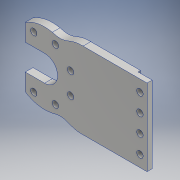
# Autodesk Inventor part: test_side_u64
Saved by Autodesk Inventor 2018 (Build 220112000, 112)
## iProperties
Created: 2016-12-19
Part Number: test_side_u64
Material: Aluminum 6061
Document SubType Name: Modeling
Designer: steve
Density: 2.7 g/cm^3
Appearance: Aluminum - Flat
Mass: 8.1898 g
Surface Area: 28.0523 cm^2
Volume: 3.03326 cm^3
Vendor: Rhoban
d13: 3,000 mm
d14: 6,000 mm
d0: 30,000 mm
d1: 22,000 mm
d2: 40,000 mm
d3: 10,100 mm
d4: 30,000 mm
d5: 28,000 mm
d6: 15,000 mm
d7: 12,000 mm
d8: 2,500 mm
d15: 3,000 mm
d16: 0,00 deg
d18: 6,000 ul
d19: 22,000 mm
d20: 225,00 deg
d22: 2,500 mm
d29: 3,000 mm
d30: 4,500 mm
d31: 4,000 ul
d33: 7,000 mm
d38: 2,500 mm
d47: 5,500 mm
d48: 1,000 mm
d49: 0,00 deg
d50: 3,100 mm
d51: 2,500 mm
d52: 1,000 mm
d53: 0,00 deg
d54: 1,500 mm
d55: 30,000 mm
d56: 7,000 mm
d57: 7,000 mm
d58: 7,000 mm
d59: 4,500 mm
d61: 2,500 mm
d68: 22,50 deg
d9: 30,000 mm
d10: 22,000 mm
d11: 21,000 mm
horn_radius_clearance: 10,100 mm
d21: 22,000 mm
d60: 4,500 mm
Author: steve
Autodesk Inventor part; units mm, degrees
ref_plane "YZ Plane" through (0, 0, 0) normal (1, 0, 0) x (0, 1, 0)
ref_plane "XZ Plane" through (0, 0, 0) normal (0, 1, 0) x (-1, 0, 0)
sketch "Sketch1" plane through (0, 0, 0) normal (0, 1, 0) x (-1, 0, 0)
  line L0 (-40, 15) -> (0, 15) construction
  line L1 (15, 15) -> (15, -15) construction
  line L2 (15, -15) -> (0, -15) construction
  line L3 (-40, -15) -> (-40, 15)
  line L4 (15, 0) -> (-40, 0) construction
  line L5 (-28.4, 0) -> (23.4, 0) construction
  circle A0 centre (0, 0) radius 11 construction
  line L6 (11, 15) -> (11, -15) construction
  circle A1 centre (0, 0) radius 5.05 construction
  line L7 (0, 5.05) -> (7.55, 5.05) construction
  line L8 (0, -5.05) -> (7.55, -5.05) construction
  line L9 (15, 15) -> (15, 5) construction
  line L10 (15, -5) -> (15, -15) construction
  arc A2 (0, 5.05) -> (0, -5.05) centre (0, 0) ccw
  circle A3 centre (0, 0) radius 15 construction
  arc A4 (0, -15) -> (14.1421, -5) centre (0, 0) ccw construction
  arc A5 (14.1421, 5) -> (0, 15) centre (0, 0) ccw construction
  line L11 (0, -15) -> (-40, -15) construction
  line L12 (0, 15) -> (15, 15) construction
  arc A6 (11, -8.6603) -> (11, 8.6603) centre (0, 0) ccw construction
  line L13 (-3, -15) -> (-3, 15) construction
  arc A7 (-3, -13.6748) -> (7.55, -11.7897) centre (0, 0) ccw
  line L14 (7.55, 5.05) -> (0, 5.05)
  line L15 (-15, -18.6523) -> (-15, 18.2394) construction
  line L16 (-40, -15) -> (-15, -15)
  line L17 (-40, 15) -> (-15, 15)
  spline S0 degree 4 poles (-3, -13.6748) (-4.5129, -13.3429) (-7.4407, -12.2328) (-10.459, -15) (-13.4863, -15) (-15, -15) knots 0 0 0 0 0 0.5 1 1 1 1 1
  spline S1 degree 4 poles (-3, 13.6748) (-4.5129, 13.3429) (-7.4407, 12.2328) (-10.459, 15) (-13.4863, 15) (-15, 15) knots 0 0 0 0 0 0.5 1 1 1 1 1
  line L18 (5.05, -15) -> (5.05, 15) construction
  line L19 (7.55, -11.7897) -> (7.55, -5.05)
  line L20 (7.55, 5.05) -> (7.55, 11.7897)
  line L21 (7.55, -5.05) -> (11, -5.05) construction
  line L22 (7.55, 5.05) -> (9.7723, 5.05) construction
  arc A8 (7.55, 11.7897) -> (7.55, -11.7897) centre (0, 0) ccw construction
  arc A9 (7.55, 11.7897) -> (-3, 13.6748) centre (0, 0) ccw
  line L23 (0, -5.05) -> (7.55, -5.05)
  line L24 (0, -26.0306) -> (0, 25.6178) construction
  line L25 (35.28, 0) -> (-47.88, 0) construction
  point P0 (13.0767, -5)
  dimension "d1" = 22
  dimension "d0" = 30
  dimension "d2" = 40
  dimension "d3" = 10.1
  dimension "d4" = 30
  dimension "d5" = 28
  dimension "d6" = 15
  dimension "d7" = 12
  dimension "d8" = 2.5
  constraints: 48 end point, 20 point on circle, 20 point on line, 9 centre point, 8 coincident, 6 collinear, 6 horizontal, 6 perpendicular, 5 parallel, 5 tangent, 5 vertical, 2 midpoint, 8 other
  measures "d0" distance of L9.start L2.start
  measures "d2" distance from line of point (0, 0) L3
  measures "d3" diameter of A1
  measures "d4" diameter of A3
  measures "d5" diameter of A6
  measures "d6" distance from line of L15 point (0, 0)
  measures "d7" distance between parallel lines of L13 L15
  measures "d8" distance between parallel lines of L19 L18
extrude "Extrusion1" add sketch "Sketch1" along normal blind 3
sketch "Sketch2" plane through (0, 3, 0) normal (0, 1, 0) x (1, 0, 0)
  circle A0 centre (0, 0) radius 11 construction
  line L0 (-21.2, 0) -> (50.2, 0) construction
  line L1 (0, 21) -> (0, -21) construction
  line L2 (0, 0) -> (-4.2095, -10.1627) construction
  point P0 (-4.2095, -10.1627)
  point P1 (4.2095, -10.1627)
  point P2 (10.1627, -4.2095)
  point P3 (10.1627, 4.2095)
  point P4 (4.2095, 10.1627)
  point P5 (-4.2095, 10.1627)
  dimension "d19" = 22
  dimension "d20" = 225
  dimension "d68" = 22.5
  constraints: 3 coincident, 2 end point, 2 point on circle, 1 centre point, 6 other
  measures "d19" diameter of A0
  measures "d68" angle of L1 L2
hole "Hole1" at (-4.2095, 3, 10.1627) at (-4.2095, 3, -10.1627) at (4.2095, 3, -10.1627) at (10.1627, 3, -4.2095) at (10.1627, 3, 4.2095) at (4.2095, 3, 10.1627) direction (0, -1, 0) diameter 2.5 end through all
sketch "Sketch3" plane through (0, 3, 0) normal (0, 1, 0) x (1, 0, 0)
  circle A0 centre (-4.2095, -10.1627) radius 1.25 construction
  circle A1 centre (4.2095, -10.1627) radius 1.25 construction
  circle A2 centre (10.1627, -4.2095) radius 1.25 construction
  circle A3 centre (10.1627, 4.2095) radius 1.25 construction
  circle A4 centre (4.2095, 10.1627) radius 1.25 construction
  circle A5 centre (-4.2095, 10.1627) radius 1.25 construction
  point P0 (0, 0)
sketch "Sketch4" plane through (0, 3, 0) normal (0, 1, 0) x (1, 0, 0)
  line L0 (37, -21.9283) -> (37, 20.7608) construction
  line L1 (40, -15) -> (40, 15) construction
  line L2 (15, -15) -> (40, -15) construction
  point P0 (0, 0)
  point P1 (37, -10.5)
  point P2 (37, -3.5)
  point P3 (37, 3.5)
  point P4 (37, 10.5)
  dimension "d29" = 3
  dimension "d30" = 4.5
  dimension "d33" = 7
  constraints: 2 end point, 2 vertical, 1 point on line, 3 other
  measures "d29" distance between parallel lines of L1 L0
  measures "d30" distance from line of L2 point (37, -10.5)
  measures "d33" distance of point (37, -10.5) point (37, -3.5)
hole "Hole2" [suppressed]
sketch "Sketch6" plane through (0, 3, 0) normal (0, 1, 0) x (1, 0, 0)
  line L0 (15, -15) -> (40, -15) projected
  line L1 (40, -15) -> (34.5, -15)
  line L2 (34.5, -15) -> (34.5, 15)
  line L3 (34.5, 15) -> (40, 15)
  line L4 (40, 15) -> (40, -15)
  line L5 (37.25, 15) -> (37.25, -15) construction
  point P0 (0, 0)
  point P1 (37.25, -10.5)
  point P2 (37.25, -3.5)
  point P3 (37.25, 3.5)
  point P4 (37.25, 10.5)
  dimension "d47" = 5.5
  dimension "d55" = 30
  dimension "d56" = 7
  dimension "d57" = 7
  dimension "d58" = 7
  dimension "d59" = 4.5
  dimension "d60" = 4.5
  constraints: 10 end point, 5 point on line, 3 midpoint, 3 parallel, 1 horizontal, 1 perpendicular
  measures "d47" distance between parallel lines of L2 L4
  measures "d55" distance between parallel lines of L3 L0
  measures "d56" distance of point (37.25, -3.5) point (37.25, -10.5)
  measures "d57" distance of point (37.25, 3.5) point (37.25, -3.5)
  measures "d58" distance of point (37.25, 3.5) point (37.25, 10.5)
  measures "d59" distance from line of L0 point (37.25, -10.5)
  measures "d60" distance from line of L3 point (37.25, 10.5)
extrude "Extrusion2" cut sketch "Sketch6" against normal blind 1
sketch "Sketch7" plane through (0, 3, 0) normal (0, 1, 0) x (1, 0, 0)
  line L0 (34.5, -15) -> (34.5, 15) projected
  line L1 (34.5, 15) -> (15, 15) projected
  arc A0 (3, 13.6748) -> (-7.55, 11.7897) centre (0, 0) ccw projected
  line L2 (-7.55, 11.7897) -> (-7.55, 5.05) projected
  line L3 (-7.55, 5.05) -> (0, 5.05) projected
  arc A1 (0, -5.05) -> (0, 5.05) centre (0, 0) ccw projected
  line L4 (0, -5.05) -> (-7.55, -5.05) projected
  line L5 (-7.55, -5.05) -> (-7.55, -11.7897) projected
  arc A2 (-7.55, -11.7897) -> (3, -13.6748) centre (0, 0) ccw projected
  line L6 (15, -15) -> (34.5, -15) projected
  circle A3 centre (10.1627, -4.2095) radius 1.25 projected
  circle A4 centre (4.2095, 10.1627) radius 1.25 projected
  circle A5 centre (-4.2095, -10.1627) radius 1.25 projected
  circle A6 centre (-4.2095, 10.1627) radius 1.25 projected
  circle A7 centre (10.1627, 4.2095) radius 1.25 projected
  circle A8 centre (4.2095, -10.1627) radius 1.25 projected
  line L7 (34.5, 1.55) -> (32, 1.55)
  line L8 (32, 1.55) -> (32, -1.55)
  line L9 (32, -1.55) -> (34.5, -1.55)
  line L10 (34.5, 0) -> (32, 0) construction
  point P0 (0, 0)
  dimension "d50" = 3.1
  dimension "d51" = 2.5
  constraints: 8 end point, 2 horizontal, 2 midpoint, 2 perpendicular, 2 point on line, 2 other
  measures "d50" distance between parallel lines of L9 L7
  measures "d51" distance of L8.end L9.end
extrude "Extrusion3" cut sketch "Sketch7" against normal blind 1 contours L9 L8 L7 L0
fillet "Fillet1" radius 1.5 2 edges at (32, 2.5, 1.55) (32, 2.5, -1.55)
hole "Hole3" at (37.25, 3, -10.5) at (37.25, 3, -3.5) at (37.25, 3, 3.5) at (37.25, 3, 10.5) direction (0, -1, 0) diameter 2.5 end through all
ref_plane "Work Plane1" through (45, 0, 15) normal (1, 0, 0) x (0, 0, -1)
equation "\"d2\" = base_2_axis"
equation "\"d3\" = horn_radius_clearance"
equation "\"d19\" = d21"
equation "\"d47\" = base_border_height"
equation "\"d9\" = 30"
equation "\"d10\" = 22"
equation "\"horn_radius_clearance\" = 10.1"
equation "\"d14\" = 2 * d13"
equation "\"d21\" = 22"
equation "\"base_2_axis\" = 40"
equation "\"base_border_height\" = 5.5"
equation "\"d13\" = 3"
body "Solid1"
